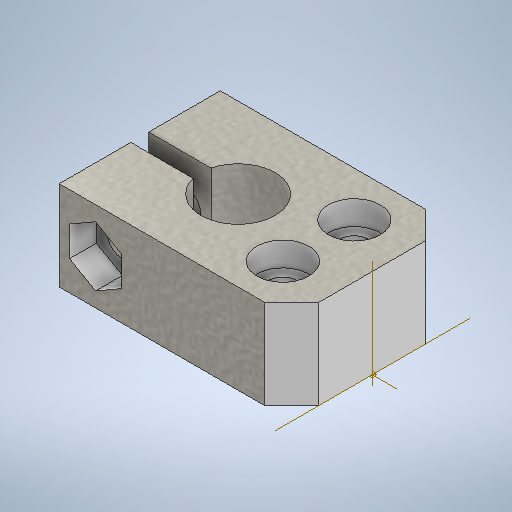
# Autodesk Inventor part: Shaft support
Saved by Autodesk Inventor 2025.2 (Build 292293000, 293)
## iProperties
Created: 2025-01-25
Part Number: Shaft support
Material: Generic
Document SubType Name: Modeling
Designer: caomi
Density: 1 g/cm^3
Appearance: Default
Author: caomi
Autodesk Inventor part; units mm, degrees
ref_plane "YZ Plane" through (0, 0, 0) normal (1, 0, 0) x (0, 1, 0)
ref_plane "XZ Plane" through (0, 0, 0) normal (0, 1, 0) x (-1, 0, 0)
ref_plane "XY Plane" through (0, 0, 0) normal (0, 0, 1) x (1, 0, 0)
sketch "Sketch1" plane through (0, 0, 0) normal (0, 1, 0) x (-1, 0, 0)
  line L0 (10.85, 0) -> (0, 0)
  line L1 (0, -9) -> (26, -9)
  line L2 (26, -9) -> (26, -1)
  circle A0 centre (15, 0) radius 4.15
  line L3 (19.0277, -1) -> (26, -1)
  line L4 (0, 9) -> (26, 9)
  line L5 (26, 9) -> (26, 1)
  circle A1 centre (15, 0) radius 4.15
  line L6 (19.0277, 1) -> (26, 1)
  line L7 (0, -9) -> (0, 0)
  line L8 (0, 9) -> (0, 0)
  point P0 (19.0277, 1)
  dimension "d2" = 1
  dimension "d3" = 9
  dimension "d4" = 8.3
  dimension "d27" = 15
  dimension "d28" = 26
  constraints: 18 end point, 4 symmetric about line, 2 horizontal, 2 point on circle, 2 point on line, 1 centre point, 1 line through centre, 1 perpendicular, 1 vertical, 3 other
  measures "d2" distance between parallel lines of L3 L0
  measures "d3" distance between parallel lines of L1 L0
  measures "d4" diameter of A0
  measures "d27" distance from line of L7 A0.centre
  measures "d28" distance between parallel lines of L7 L2
extrude "Extrusion1" add sketch "Sketch1" along normal blind 10 contours A0 L3 L2 L1 L7 L0 | L0 L8 L4 L5 L6 A0
sketch "Sketch7" plane through (0, 10, 0) normal (0, 1, 0) x (1, 0, 0)
  line L0 (0, -9) -> (0, 9) projected
  line L1 (-31.2, 0) -> (5.2, 0) projected
  arc A0 (-19.0277, -1) -> (-19.0277, 1) centre (-15, 0) ccw projected
  point P0 (0, 0)
  point P1 (-6, -4)
  point P2 (0, 0)
  point P3 (-6, 4)
  dimension "d44" = 8
  dimension "d45" = 9
  constraints: 1 midpoint, 1 symmetric about line, 1 vertical alignment
  measures "d44" distance of point (-6, 4) point (-6, -4)
  measures "d45" horizontal distance of A0.centre point (-6, 4)
hole "Hole1" at (-6, 10, 4) at (-6, 10, -4) direction (0, -1, 0) diameter 3.3 end through all counterbore diameter 5.8 counterbore depth 2.7
sketch "Sketch3" plane through (0, 0, -9) normal (0, 0, -1) x (-1, 0, 0)
  circle A0 centre (21.9389, 5) radius 1.75
  line L0 (26, 0) -> (26, 10) projected
  line L1 (10.85, 10) -> (19.0277, 10) projected
  point P0 (0, 0)
  point P1 (26, 5)
  point P2 (14.9389, 10)
  dimension "d15" = 3.5
  dimension "d46" = 7
  constraints: 2 midpoint, 1 centre point, 1 horizontal alignment
  measures "d15" diameter of A0
  measures "d46" horizontal distance of point (14.939, 10) A0.centre
extrude "Extrusion3" cut sketch "Sketch3" against normal up to surface (18 mm away)
sketch "Sketch4" plane through (-26, 0, 9) normal (0, 0, 1) x (1, 0, 0)
  line L0 (1.1611, 6.6743) -> (4.0611, 8.3486)
  line L1 (4.0611, 8.3486) -> (6.9611, 6.6743)
  line L2 (6.9611, 6.6743) -> (6.9611, 3.3257)
  line L3 (6.9611, 3.3257) -> (4.0611, 1.6514)
  line L4 (4.0611, 1.6514) -> (1.1611, 3.3257)
  line L5 (1.1611, 3.3257) -> (1.1611, 6.6743)
  circle A0 centre (4.0611, 5) radius 1.75 projected
  point P0 (26, 0)
  point P1 (1.1611, 5)
  dimension "d20" = 5.8
  constraints: 12 end point, 1 coincident, 1 midpoint, 1 vertical, 13 other
  measures "d20" distance from line of L2 point (1.161, 5)
extrude "Extrusion4" cut sketch "Sketch4" against normal blind 3
sketch "Sketch5" plane through (0, 0, -9) normal (0, 0, -1) x (-1, 0, 0)
  circle A0 centre (21.9389, 5) radius 2.9
  circle A1 centre (21.9389, 5) radius 1.75 projected
  point P0 (0, 0)
  dimension "d23" = 5.8
  constraints: 1 centre point, 1 coincident
  measures "d23" diameter of A0
extrude "Extrusion5" cut sketch "Sketch5" against normal blind 2
chamfer "Chamfer1" distance 3 angle 45 2 edges at (0, 5, 9) (0, 5, -9)
equation "\"d17\" = d15"
body "Solid1"
